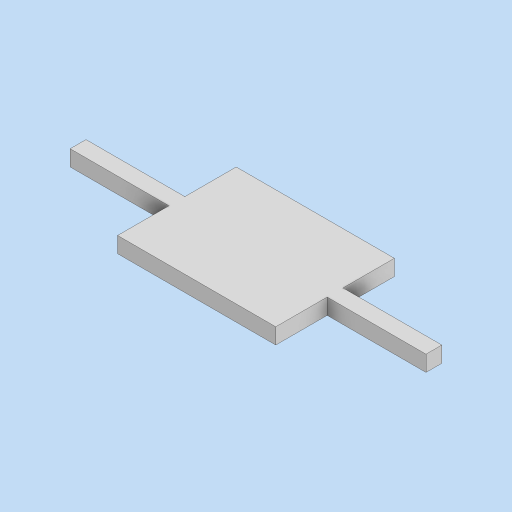
# Autodesk Inventor part: BASE_DE_PRUEBA
Saved by Autodesk Inventor 2024 (Build 280153000, 153)
## iProperties
Created: 2024-10-01
Part Number: BASE_DE_PRUEBA
Material: Generic
Document SubType Name: Modeling
Designer: MxMon
Density: 1 g/cm^3
Appearance: Default
Author: MxMon
Autodesk Inventor part; units mm, degrees
ref_plane "YZ Plane" through (0, 0, 0) normal (1, 0, 0) x (0, 1, 0)
ref_plane "XZ Plane" through (0, 0, 0) normal (0, 1, 0) x (-1, 0, 0)
ref_plane "XY Plane" through (0, 0, 0) normal (0, 0, 1) x (1, 0, 0)
sketch "Sketch1" plane through (0, 0, 0) normal (0, 1, 0) x (-1, 0, 0)
  line L0 (31.25, 5) -> (-31.25, 5)
  line L1 (-31.25, 5) -> (-31.25, -5)
  line L2 (-31.25, -5) -> (31.25, -5)
  line L3 (31.25, -5) -> (31.25, 5)
  line L4 (31.25, 5) -> (-31.25, -5) construction
  line L5 (-31.25, 5) -> (31.25, -5) construction
  line L6 (31.25, -37.5) -> (131.25, -37.5)
  line L7 (131.25, -37.5) -> (131.25, 37.5)
  line L8 (131.25, 37.5) -> (31.25, 37.5)
  line L9 (31.25, 37.5) -> (31.25, -37.5)
  line L10 (131.25, -5) -> (193.75, -5)
  line L11 (193.75, -5) -> (193.75, 5)
  line L12 (193.75, 5) -> (131.25, 5)
  line L13 (131.25, 5) -> (131.25, -5)
  point P0 (0, 0)
  point P1 (31.25, 0)
  point P2 (193.75, 0)
  point P3 (131.25, 0)
  point P4 (131.25, 5)
  point P5 (31.25, 5)
  point P6 (31.25, -5)
  dimension "d0" = 62.5
  dimension "d1" = 10
  dimension "d2" = 75
  dimension "d3" = 100
  constraints: 28 end point, 6 midpoint, 6 parallel, 3 horizontal, 3 perpendicular, 2 equal length, 1 horizontal alignment, 1 point on line
  measures "d0" distance of L2.end L1.end
  measures "d1" distance of L0.end L1.end
  measures "d2" distance of L6.end L7.end
  measures "d3" distance of L6.start L6.end
extrude "Extrusion1" add sketch "Sketch1" along normal blind 10
body "Solid1"
